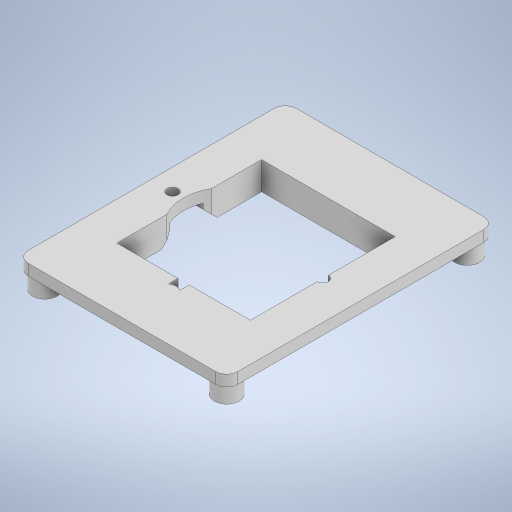
# Autodesk Inventor part: ServoFullMountInsert
Saved by Autodesk Inventor 2024.2 (Build 282272000, 272)
## iProperties
Created: 2024-04-03
Part Number: ServoFullMountInsert
Material: Generic
Document SubType Name: Modeling
Designer: ringl
Density: 1 g/cm^3
Appearance: Default
Author: ringl
Autodesk Inventor part; units mm, degrees
ref_plane "YZ Plane" through (0, 0, 0) normal (1, 0, 0) x (0, 1, 0)
ref_plane "XZ Plane" through (0, 0, 0) normal (0, 1, 0) x (-1, 0, 0)
ref_plane "XY Plane" through (0, 0, 0) normal (0, 0, 1) x (1, 0, 0)
sketch "Sketch1" plane through (0, 0, 0) normal (0, 1, 0) x (-1, 0, 0)
  line L0 (0, 0) -> (28, 0)
  line L1 (28, 0) -> (28, -38.5)
  line L2 (28, -38.5) -> (0, -38.5)
  line L3 (0, -38.5) -> (0, 0)
  line L4 (26, -6.25) -> (2, -6.25)
  line L5 (2, -6.25) -> (2, -32.25)
  line L6 (2, -32.25) -> (26, -32.25)
  line L7 (26, -32.25) -> (26, -6.25)
  dimension "d0" = 28
  dimension "d1" = 38.5
  dimension "d2" = 24
  dimension "d3" = 26
  dimension "d43" = 2
  dimension "d44" = 6.25
  constraints: 16 end point, 4 parallel, 2 horizontal, 2 perpendicular
  measures "d0" distance of L1.end L2.end
  measures "d1" distance of L0.end L1.end
  measures "d2" distance of L6.end L5.end
  measures "d3" distance of L5.end L4.end
  measures "d43" distance between parallel lines of L3 L5
  measures "d44" distance between parallel lines of L2 L6
extrude "Extrusion1" add sketch "Sketch1" along normal blind 3
sketch "Sketch2" plane through (0, 3, 0) normal (0, 1, 0) x (1, 0, 0)
  line L0 (-28, 0) -> (0, 0) projected
  circle A0 centre (0, 0) radius 2
  circle A1 centre (-28, 0) radius 2
  line L1 (0, 38.5) -> (-28, 38.5) projected
  circle A2 centre (-28, 38.5) radius 2
  circle A3 centre (0, 38.5) radius 2
  dimension "d8" = 4
  dimension "d9" = 4
  dimension "d10" = 4
  dimension "d11" = 4
  constraints: 4 centre point, 3 coincident
  measures "d8" diameter of A0
  measures "d9" diameter of A1
  measures "d10" diameter of A2
  measures "d11" diameter of A3
extrude "Extrusion2" cut sketch "Sketch2" against normal blind 3
sketch "Sketch3" plane through (0, 3, 0) normal (0, 1, 0) x (1, 0, 0)
  line L0 (-32.85, 43.35) -> (4.85, 43.35)
  line L1 (4.85, 43.35) -> (4.85, -4.85)
  line L2 (4.85, -4.85) -> (-32.85, -4.85)
  line L3 (-32.85, -4.85) -> (-32.85, 43.35)
  line L4 (-2, 38.5) -> (-26, 38.5) projected
  line L5 (0, 2) -> (0, 36.5) projected
  line L6 (-2, 32.25) -> (-2, 6.25) projected
  line L7 (-26, 6.25) -> (-26, 32.25) projected
  line L8 (-2, 6.25) -> (-26, 6.25)
  line L9 (-26, 6.25) -> (-26, 32.25)
  line L10 (-26, 32.25) -> (-2, 32.25)
  line L11 (-2, 32.25) -> (-2, 6.25)
  point P0 (0, 0)
  point P1 (-26, 6.25)
  dimension "d14" = 48.2
  dimension "d15" = 37.7
  dimension "d16" = 4.85
  dimension "d17" = 4.85
  constraints: 16 end point, 4 parallel, 2 horizontal, 2 perpendicular
  measures "d14" distance of L0.end L1.end
  measures "d15" distance of L1.end L2.end
  measures "d16" distance between parallel lines of L0 L4
  measures "d17" distance between parallel lines of L5 L1
extrude "Extrusion3" add sketch "Sketch3" along normal blind 2
sketch "Sketch4" plane through (0, 3, 0) normal (0, -1, 0) x (1, 0, 0)
  circle A0 centre (2.35, -40.85) radius 2.25
  line L0 (-2, -38.5) -> (-26, -38.5) projected
  line L1 (0, -2) -> (0, -36.5) projected
  circle A1 centre (-30.35, -40.85) radius 2.25
  line L2 (-28, -36.5) -> (-28, -2) projected
  circle A2 centre (-30.35, 2.35) radius 2.25
  line L3 (-26, 0) -> (-2, 0) projected
  circle A3 centre (2.35, 2.35) radius 2.25
  point P0 (0, 0)
  dimension "d20" = 4.5
  dimension "d21" = 2.35
  dimension "d22" = 2.35
  dimension "d23" = 4.5
  dimension "d24" = 2.35
  dimension "d25" = 2.35
  dimension "d26" = 4.5
  dimension "d27" = 2.35
  dimension "d28" = 4.5
  dimension "d29" = 2.35
  dimension "d30" = 2.35
  dimension "d31" = 2.35
  constraints: 4 centre point
  measures "d20" diameter of A0
  measures "d21" distance from line of A0.centre L0
  measures "d22" distance from line of A0.centre L1
  measures "d23" diameter of A1
  measures "d24" distance from line of L2 A1.centre
  measures "d25" distance from line of L0 A1.centre
  measures "d26" diameter of A2
  measures "d27" distance from line of L3 A2.centre
  measures "d28" diameter of A3
  measures "d29" distance from line of L1 A3.centre
  measures "d30" distance from line of L3 A3.centre
  measures "d31" distance from line of L2 A2.centre
extrude "Extrusion4" add sketch "Sketch4" along normal blind 3
fillet "Fillet1" radius 2 4 edges at (4.85, 4, -43.35) (4.85, 4, 4.85) (-32.85, 4, 4.85) (-32.85, 4, -43.35)
sketch "Sketch5" plane through (0, 5, 0) normal (0, 1, 0) x (1, 0, 0)
  line L0 (-26, 32.25) -> (-2, 32.25) projected
  line L1 (-2, 6.25) -> (-26, 6.25) projected
  line L2 (-2, 32.25) -> (-2, 6.25) projected
  line L3 (-26, 6.25) -> (-26, 32.25) projected
  circle A0 centre (-2, 19.25) radius 1
  circle A1 centre (-29, 19.25) radius 1
  line L4 (4.85, -2.85) -> (4.85, 41.35) projected
  point P0 (0, 0)
  dimension "d45" = 2
  dimension "d46" = 2
  dimension "d47" = 13
  dimension "d50" = 13
  dimension "d73" = 27
  dimension "d75" = 3
  constraints: 2 centre point
  measures "d45" diameter of A0
  measures "d46" diameter of A1
  measures "d47" distance from line of L1 A1.centre
  measures "d50" distance from line of L0 A0.centre
  measures "d73" distance of A1.centre A0.centre
  measures "d75" distance from line of L3 A1.centre
extrude "Extrusion6" cut sketch "Sketch5" against normal through all contours A0 L2 | L2 A0 | A1
sketch "Sketch6" plane through (-28, 0, -36.5) normal (-1, 0, 0) x (0, 0, 1)
  line L0 (0, 0) -> (34.5, 0) projected
  line L1 (-4.85, 3) -> (39.35, 3) projected
  line L2 (20.25, 0) -> (14.25, 0)
  line L3 (14.25, 0) -> (14.25, 3)
  line L4 (14.25, 3) -> (20.25, 3)
  line L5 (20.25, 3) -> (20.25, 0)
  line L6 (41.35, 3) -> (41.35, 5) projected
  point P0 (36.5, 0)
  point P1 (41.35, 4)
  dimension "d53" = 6
  dimension "d54" = 21.1
  constraints: 8 end point, 2 parallel, 2 point on line, 1 horizontal, 1 midpoint, 1 perpendicular
  measures "d53" distance between parallel lines of L3 L5
  measures "d54" distance from line of point (41.35, 4) L5
extrude "Extrusion7" cut sketch "Sketch6" against normal blind 10
chamfer "Chamfer1" distance 2 angle 45 2 edges at (-27, 0, -22.25) (-27, 0, -16.25)
sketch "Sketch7" plane through (0, 5, 0) normal (0, 1, 0) x (1, 0, 0)
  line L0 (-30.85, -4.85) -> (2.85, -4.85) projected
  line L1 (-26, 6.25) -> (-26, 32.25) projected
  arc A0 (-26, 23.25) -> (-26, 15.25) centre (-19.0718, 19.25) ccw
  line L2 (-26, 23.25) -> (-26, 15.25)
  point P0 (0, 0)
  dimension "d63" = 8
  dimension "d64" = 20.1
  dimension "d65" = 8
  constraints: 2 end point, 2 point on circle, 2 point on line, 1 centre point, 1 vertical
  measures "d63" distance of L2.start L2.end
  measures "d64" distance from line of L0 L2.end
  measures "d65" radius of A0
extrude "Extrusion8" cut sketch "Sketch7" against normal blind 10
sketch "Sketch8" plane through (0, 5, 0) normal (0, 1, 0) x (1, 0, 0)
  circle A0 centre (-14, 3.125) radius 1.75
  line L0 (-2, 6.25) -> (-26, 6.25) projected
  line L1 (-26, 0) -> (-2, 0) projected
  line L2 (-32.85, 41.35) -> (-32.85, -2.85) projected
  point P0 (0, 0)
  dimension "d68" = 3.5
  dimension "d69" = 3.125
  dimension "d70" = 18.85
  constraints: 1 centre point
  measures "d68" diameter of A0
  measures "d69" distance from line of L1 A0.centre
  measures "d70" distance from line of L2 A0.centre
extrude "Extrusion9" [suppressed]
sketch "Sketch9" plane through (0, 5, 0) normal (0, 1, 0) x (1, 0, 0)
  circle A0 centre (-14, 3.125) radius 1.75 projected
  line L0 (-15, 4.5611) -> (-15, 6.25)
  line L1 (-15, 6.25) -> (-13, 6.25)
  line L2 (-13, 6.25) -> (-13, 4.5611)
  arc A1 (-13, 4.5611) -> (-15, 4.5611) centre (-14, 3.125) ccw
  line L3 (-2, 6.25) -> (-26, 6.25) projected
  point P0 (0, 0)
  point P1 (-14, 6.25)
  dimension "d76" = 2
  dimension "d77" = 1
  constraints: 6 end point, 4 point on circle, 2 midpoint, 2 perpendicular, 1 centre point, 1 concentric, 1 vertical
  measures "d76" distance of L0.end L1.end
  measures "d77" distance from line of A0.centre L2
extrude "Extrusion10" cut sketch "Sketch9" against normal through all contours A0 L0 L1 L2
fillet "Fillet2" [suppressed]
body "Solid1"
